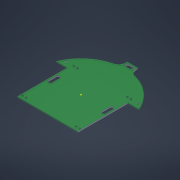
# Autodesk Inventor part: flame
Saved by Autodesk Inventor 2022 (Build 260153000, 153)
## iProperties
Created: 2021-09-22
Part Number: flame
Material: エポキシ樹脂
Document SubType Name: Modeling
Designer: shiok
Density: 1.14 g/cm^3
Appearance: 透明 - スレート 青
Author: shiok
Autodesk Inventor part; units mm, degrees
ref_plane "YZ Plane" through (0, 0, 0) normal (1, 0, 0) x (0, 1, 0)
ref_plane "XZ Plane" through (0, 0, 0) normal (0, 1, 0) x (-1, 0, 0)
ref_plane "XY Plane" through (0, 0, 0) normal (0, 0, 1) x (1, 0, 0)
sketch "スケッチ1" plane through (0, 0, 0) normal (0, 1, 0) x (-1, 0, 0)
  circle A0 centre (0, 0) radius 62.5
  line L0 (62.5, 0) -> (-62.5, 0)
  line L1 (-62.5, 0) -> (-62.5, 47)
  line L2 (-62.5, 47) -> (62.5, 47)
  line L3 (62.5, 47) -> (62.5, 0)
  line L4 (53.7658, -31.8667) -> (53.7658, -24.7446)
  line L5 (53.7658, -24.7446) -> (57.393, -24.7446)
  line L6 (0, -62.5) -> (0, -72.5)
  line L7 (0, -72.5) -> (7.5, -72.5)
  line L8 (7.5, -72.5) -> (7.5, -62.0484)
  line L9 (0, -72.5) -> (-7.5, -72.5)
  line L10 (-7.5, -72.5) -> (-7.5, -62.0484)
  point P0 (41.1977, 47)
  point P1 (3.75, -60.165)
  point P2 (-3.75, -60.165)
  point P3 (-41.1977, 47)
  dimension "d41" = 125
  dimension "d70" = 60.165
  dimension "d71" = 7.5
  dimension "d72" = 3.75
  dimension "d88" = 47
  dimension "d102" = 7.5
  dimension "d103" = 10
  constraints: 22 end point, 4 parallel, 2 perpendicular, 2 vertical, 1 coincident, 1 collinear, 1 horizontal, 1 horizontal alignment, 1 midpoint, 1 point on line, 1 symmetric about line, 10 other
  measures "d70" vertical distance of point (3.75, -60.165) point (0, 0)
  measures "d71" distance of point (-3.75, -60.165) point (3.75, -60.165)
  measures "d72" horizontal distance of point (0, 0) point (3.75, -60.165)
  measures "d88" distance between parallel lines of L0 L2
  measures "d102" distance of L7.end L6.end
  measures "d103" distance of L6.end L6.start
extrude "押し出し1" add sketch "スケッチ1" along normal blind 1.6 contours L0 A0 L5 L4 | L1 L2 A0 | A0 L2 L0 | A0 L6 L9 L10 | A0 L2 L3 | A0 L8 L7 L6 | A0 L4 L5
sketch "スケッチ6" plane through (0, 1.6, 0) normal (0, 1, 0) x (-1, 0, 0)
  line L0 (-35, -30) -> (-35, 42) construction
  line L1 (-35, 42) -> (-40, 42) construction
  line L2 (-40, 42) -> (-40, -30) construction
  line L3 (-35, 12) -> (-40, 12) construction
  line L4 (-42.5, 21.5) -> (-42.5, -18.5) construction
  line L5 (-35, -30) -> (-40, -30) construction
  line L6 (-42.5, 20) -> (-42.5, -20) construction
  point P0 (0, 0)
  point P1 (-37.5, 0)
  dimension "d52" = 5
  dimension "d53" = 72
  dimension "d54" = 30
  dimension "d55" = 2.5
  dimension "d68" = 35
  dimension "d69" = 12
  dimension "d100" = 30
  constraints: 14 end point, 2 point on line, 1 horizontal, 1 parallel, 1 perpendicular
  measures "d52" distance of L1.end L0.end
  measures "d53" distance of L0.end L0.start
  measures "d54" distance between parallel lines of L1 L3
  measures "d55" distance between parallel lines of L2 L4
  measures "d68" distance from line of point (0, 0) L0
  measures "d69" distance from line of point (0, 0) L3
  measures "d100" distance from line of L5 point (-37.5, 0)
hole "穴3" at (35, 1.6, 42) at (40, 1.6, 42) at (40, 1.6, -30) at (35, 1.6, -30) at (37.5, 1.6, 0) direction (0, -1, 0) diameter 2.4 end through all clearance for "Countersunk Flat Head Screw ISO 2009/7046" size "M2" standard "ISO"
mirror "ミラー2" about plane through (0, 0, 0) normal (1, 0, 0) of "穴3"
sketch "スケッチ9" plane through (0, 1.6, 0) normal (0, 1, 0) x (1, 0, 0)
  line L0 (-42.5, 23) -> (-72.5, 23)
  line L1 (-72.5, 23) -> (-72.5, -32)
  line L2 (-72.5, -32) -> (-42.5, -32)
  line L3 (-42.5, -32) -> (-42.5, 23)
  line L4 (-62.5, 0) -> (-62.5, -47) projected
  line L5 (-62.5, -47) -> (62.5, -47) projected
  line L6 (-42.5, -32) -> (-72.5, -32)
  line L7 (-72.5, -32) -> (-72.5, -49)
  line L8 (-72.5, -49) -> (-42.5, -49)
  line L9 (-42.5, -49) -> (-42.5, -32)
  point P0 (0, 0)
  point P1 (-42.5, -47)
  point P2 (-62.5, -32)
  dimension "d84" = 55
  dimension "d89" = 23
  dimension "d90" = 42.5
  dimension "d91" = 30
  dimension "d92" = 17
  constraints: 16 end point, 4 parallel, 2 horizontal, 2 perpendicular, 1 collinear
  measures "d84" distance between parallel lines of L0 L2
  measures "d89" distance from line of L0 point (0, 0)
  measures "d90" distance from line of L3 point (0, 0)
  measures "d91" distance of L1.end L2.end
  measures "d92" distance of L7.end L6.end
extrude "押し出し2" cut sketch "スケッチ9" against normal blind 10 contours L3 L2 L1 L0 | L9 L5 L4 L2
mirror "ミラー3" about plane through (0, 0, 0) normal (1, 0, 0) of "押し出し2"
sketch "スケッチ10" plane through (0, 1.6, 0) normal (0, 1, 0) x (1, 0, 0)
  circle A0 centre (-35, 30) radius 1.2 projected
  circle A1 centre (-40, 30) radius 1.2 projected
  line L0 (-35, 30) -> (-50, 30) construction
  point P0 (0, 0)
  dimension "d101" = 15
  constraints: 2 end point, 1 coincident, 1 horizontal
  measures "d101" distance of L0.start L0.end
hole "穴5" at (-50, 1.6, -30) direction (0, -1, 0) diameter 2.4 depth 1.6 tip angle 118 clearance for "Countersunk Flat Head Screw ISO 2009/7046" size "M2" standard "ISO"
mirror "ミラー4" about plane through (0, 0, 0) normal (1, 0, 0) of "穴5"
sketch "スケッチ12" plane through (0, 1.6, 0) normal (0, 1, 0) x (1, 0, 0)
  line L0 (-56.8017, 16.1133) -> (59.6732, 16.1133) construction
  line L1 (59.6732, 16.1133) -> (59.6732, -15.1509) construction
  line L2 (59.6732, -15.1509) -> (-56.8017, -15.1509) construction
  line L3 (-56.8017, -15.1509) -> (-56.8017, 16.1133) construction
  point P0 (0, 0)
  constraints: 2 other
sketch "スケッチ13" plane through (0, 1.6, 0) normal (0, 1, 0) x (1, 0, 0)
  point P0 (0, 0)
sketch "スケッチ14" plane through (0, 0, 0) normal (0, -1, 0) x (1, 0, 0)
  line L0 (7.5, -72.5) -> (-7.5, -72.5) projected
  line L1 (0, -72.5) -> (0, -62.5192)
  point P0 (0, 0)
  point P1 (5.625, -68)
  point P2 (-5.625, -68)
  dimension "d104" = 4.5
  dimension "d106" = 11.25
  constraints: 2 end point, 1 midpoint, 1 symmetric about line, 1 vertical
  measures "d104" distance from line of L0 point (5.625, -68)
  measures "d106" distance of point (-5.625, -68) point (5.625, -68)
hole "穴6" at (5.625, 0, -68) at (-5.625, 0, -68) direction (0, 1, 0) diameter 2.4 end through all clearance for "Countersunk Flat Head Screw ISO 2009/7046" size "M2" standard "ISO"
sketch "スケッチ15" plane through (0, 0, 0) normal (0, -1, 0) x (1, 0, 0)
  line L0 (2.15, -65.75) -> (-2.15, -65.75)
  line L1 (-3.75, -67.35) -> (-3.75, -68.65)
  line L2 (-2.15, -70.25) -> (2.15, -70.25)
  line L3 (3.75, -68.65) -> (3.75, -67.35)
  arc A0 (3.75, -67.35) -> (2.15, -65.75) centre (2.15, -67.35) ccw
  arc A1 (2.15, -70.25) -> (3.75, -68.65) centre (2.15, -68.65) ccw
  arc A2 (-3.75, -68.65) -> (-2.15, -70.25) centre (-2.15, -68.65) ccw
  arc A3 (-2.15, -65.75) -> (-3.75, -67.35) centre (-2.15, -67.35) ccw
  line L4 (3.75, -68) -> (-3.75, -68)
  line L5 (0, -65.75) -> (0, -70.25)
  circle A4 centre (5.625, -68) radius 1.2 projected
  circle A5 centre (-5.625, -68) radius 1.2 projected
  point P0 (0, 0)
  point P1 (-3.75, -70.25)
  point P2 (-3.75, -65.75)
  point P3 (3.75, -70.25)
  dimension "d114" = 7.5
  dimension "d115" = 4.5
  dimension "d116" = 1.6
  constraints: 12 end point, 8 point on circle, 8 point on line, 8 tangent, 4 centre point, 4 midpoint, 3 equal radius, 2 parallel, 1 horizontal, 1 perpendicular
  measures "d114" distance of point (3.75, -70.25) point (-3.75, -70.25)
  measures "d115" distance of point (-3.75, -70.25) point (-3.75, -65.75)
  measures "d116" radius of A0
extrude "押し出し3" cut sketch "スケッチ15" against normal blind 1.6 contours A0 L3 L4 L5 L0 | L5 L4 L1 A3 L0 | L5 L2 A2 L1 L4 | L4 L3 A1 L2 L5
fillet "フィレット1" radius 10 2 edges at (7.5, 0.8, -62.0484) (-7.5, 0.8, -62.0484)
sketch "スケッチ16" plane through (0, 0, 0) normal (0, -1, 0) x (1, 0, 0)
  circle A0 centre (-37.5, 0) radius 1.2 projected
  line L0 (-35, -7.5) -> (-40, -7.5)
  line L1 (-40, -7.5) -> (-40, 7.5)
  line L2 (-40, 7.5) -> (-35, 7.5)
  line L3 (-35, 7.5) -> (-35, -7.5)
  line L4 (-35, -7.5) -> (-40, 7.5) construction
  line L5 (-35, 7.5) -> (-40, -7.5) construction
  point P0 (0, 0)
  point P1 (-37.5, 0)
  dimension "d120" = 5
  dimension "d121" = 15
  constraints: 12 end point, 3 midpoint, 2 parallel, 1 coincident, 1 horizontal, 1 perpendicular
  measures "d120" distance of L1.end L2.end
  measures "d121" distance of L0.end L1.end
extrude "押し出し4" cut sketch "スケッチ16" against normal blind 10
fillet "フィレット2" radius 2 4 edges at (-35, 0.8, -7.5) (-35, 0.8, 7.5) (-40, 0.8, 7.5) (-40, 0.8, -7.5)
mirror "ミラー5" about plane through (0, 0, 0) normal (1, 0, 0) of "押し出し4", "フィレット2"
